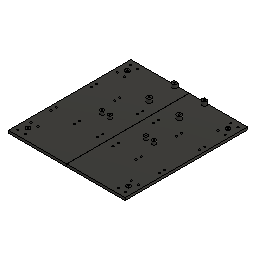
base_plate (Autodesk Fusion 360 design; units mm, degrees)
Autodesk Fusion 360 part; units mm, degrees
note: some values were not read from the file. Set by a fixed rule: which sketch regions a step uses.
sketch "Skizze2" plane through (0, 0, 0) normal (0, 0, 1) x (1, 0, 0)
  line L0 (0, 153.3528) -> (0, -137.2618) construction
  line L1 (-213.5725, 0) -> (204.3079, 0) construction
  line L2 (113.137, -118.8) -> (-113.137, -118.8)
  line L3 (-113.137, -118.8) -> (-113.137, 118.8)
  line L4 (-113.137, 118.8) -> (113.137, 118.8)
  line L5 (113.137, 118.8) -> (113.137, -118.8)
  line L6 (113.137, -118.8) -> (-113.137, 118.8) construction
  line L7 (-113.137, -118.8) -> (113.137, 118.8) construction
  line L8 (0, 118.8) -> (0, -118.8)
  line L9 (-140.8962, -96.5) -> (185.8278, -96.5) construction
  line L10 (-143.9931, -39) -> (195.1185, -39) construction
  line L11 (97.637, 133.9785) -> (97.637, -173.5851) construction
  line L12 (104.637, -109) -> (90.637, -109) construction
  line L13 (90.637, -109) -> (90.637, -84) construction
  line L14 (90.637, -84) -> (104.637, -84) construction
  line L15 (104.637, -84) -> (104.637, -109) construction
  line L16 (104.637, -109) -> (90.637, -84) construction
  line L17 (90.637, -109) -> (104.637, -84) construction
  circle A0 centre (104.637, -84) radius 1.75
  circle A1 centre (104.637, -84) radius 3.5
  circle A2 centre (90.637, -84) radius 1.75
  circle A3 centre (90.637, -84) radius 3.5
  circle A4 centre (90.637, -109) radius 1.75
  circle A5 centre (90.637, -109) radius 3.5
  circle A6 centre (104.637, -109) radius 1.75
  circle A7 centre (104.637, -109) radius 3.5
  circle A8 centre (-90.637, -109) radius 3.5
  circle A9 centre (-90.637, -109) radius 1.75
  circle A10 centre (-104.637, -109) radius 3.5
  circle A11 centre (-104.637, -109) radius 1.75
  circle A12 centre (-104.637, -84) radius 3.5
  circle A13 centre (-104.637, -84) radius 1.75
  circle A14 centre (-90.637, -84) radius 3.5
  circle A15 centre (-90.637, -84) radius 1.75
  circle A16 centre (104.637, 84) radius 3.5
  circle A17 centre (104.637, 84) radius 1.75
  circle A18 centre (90.637, 84) radius 3.5
  circle A19 centre (90.637, 84) radius 1.75
  circle A20 centre (90.637, 109) radius 3.5
  circle A21 centre (90.637, 109) radius 1.75
  circle A22 centre (104.637, 109) radius 3.5
  circle A23 centre (104.637, 109) radius 1.75
  circle A24 centre (-104.637, 109) radius 3.5
  circle A25 centre (-104.637, 109) radius 1.75
  circle A26 centre (-90.637, 109) radius 3.5
  circle A27 centre (-90.637, 109) radius 1.75
  circle A28 centre (-90.637, 84) radius 3.5
  circle A29 centre (-90.637, 84) radius 1.75
  circle A30 centre (-104.637, 84) radius 3.5
  circle A31 centre (-104.637, 84) radius 1.75
  line L18 (15, -28.2196) -> (15, -51.638) construction
  circle A32 centre (15, -34) radius 1.75
  circle A33 centre (15, -44) radius 1.75
  circle A34 centre (15, -34) radius 3.5
  circle A35 centre (15, -44) radius 3.5
  circle A36 centre (-15, -34) radius 3.5
  circle A37 centre (-15, -34) radius 1.75
  circle A38 centre (-15, -44) radius 3.5
  circle A39 centre (-15, -44) radius 1.75
  circle A40 centre (60, -34) radius 3.5
  circle A41 centre (60, -34) radius 1.75
  circle A42 centre (60, -44) radius 3.5
  circle A43 centre (60, -44) radius 1.75
  circle A44 centre (105, -34) radius 3.5
  circle A45 centre (105, -34) radius 1.75
  circle A46 centre (105, -44) radius 3.5
  circle A47 centre (105, -44) radius 1.75
  circle A48 centre (-60, -44) radius 1.75
  circle A49 centre (-60, -44) radius 3.5
  circle A50 centre (-60, -34) radius 1.75
  circle A51 centre (-60, -34) radius 3.5
  circle A52 centre (-105, -44) radius 1.75
  circle A53 centre (-105, -44) radius 3.5
  circle A54 centre (-105, -34) radius 1.75
  circle A55 centre (-105, -34) radius 3.5
  circle A56 centre (105, 44) radius 3.5
  circle A57 centre (105, 34) radius 3.5
  circle A58 centre (105, 34) radius 1.75
  circle A59 centre (60, 44) radius 3.5
  circle A60 centre (60, 44) radius 1.75
  circle A61 centre (60, 34) radius 3.5
  circle A62 centre (60, 34) radius 1.75
  circle A63 centre (15, 44) radius 3.5
  circle A64 centre (15, 44) radius 1.75
  circle A65 centre (15, 34) radius 3.5
  circle A66 centre (15, 34) radius 1.75
  circle A67 centre (-15, 34) radius 3.5
  circle A68 centre (-15, 34) radius 1.75
  circle A69 centre (-15, 44) radius 3.5
  circle A70 centre (-15, 44) radius 1.75
  circle A71 centre (-60, 44) radius 3.5
  circle A72 centre (-60, 44) radius 1.75
  circle A73 centre (-60, 34) radius 3.5
  circle A74 centre (-60, 34) radius 1.75
  circle A75 centre (-105, 34) radius 3.5
  circle A76 centre (-105, 34) radius 1.75
  circle A77 centre (-105, 44) radius 1.75
  circle A78 centre (-105, 44) radius 3.5
  circle A79 centre (97.637, -96.5) radius 1.25
  circle A80 centre (97.637, -96.5) radius 4
  line L19 (98.9072, -98.7) -> (100.1773, -96.5)
  line L20 (100.1773, -96.5) -> (98.9072, -94.3)
  line L21 (98.9072, -94.3) -> (96.3668, -94.3)
  line L22 (96.3668, -94.3) -> (95.0967, -96.5)
  line L23 (95.0967, -96.5) -> (96.3668, -98.7)
  line L24 (96.3668, -98.7) -> (98.9072, -98.7)
  circle A81 centre (97.637, 96.5) radius 4
  line L25 (96.3668, 94.3) -> (95.0967, 96.5)
  line L26 (95.0967, 96.5) -> (96.3668, 98.7)
  line L27 (96.3668, 98.7) -> (98.9072, 98.7)
  line L28 (98.9072, 98.7) -> (100.1773, 96.5)
  line L29 (98.9072, 94.3) -> (96.3668, 94.3)
  line L30 (100.1773, 96.5) -> (98.9072, 94.3)
  circle A82 centre (97.637, 96.5) radius 1.25
  circle A83 centre (-97.637, -96.5) radius 4
  line L31 (-98.9072, -94.3) -> (-96.3668, -94.3)
  line L32 (-96.3668, -94.3) -> (-95.0967, -96.5)
  line L33 (-95.0967, -96.5) -> (-96.3668, -98.7)
  line L34 (-96.3668, -98.7) -> (-98.9072, -98.7)
  line L35 (-100.1773, -96.5) -> (-98.9072, -94.3)
  line L36 (-98.9072, -98.7) -> (-100.1773, -96.5)
  circle A84 centre (-97.637, -96.5) radius 1.25
  circle A85 centre (-97.637, 96.5) radius 4
  line L37 (-95.0967, 96.5) -> (-96.3668, 98.7)
  line L38 (-96.3668, 98.7) -> (-98.9072, 98.7)
  line L39 (-98.9072, 98.7) -> (-100.1773, 96.5)
  line L40 (-100.1773, 96.5) -> (-98.9072, 94.3)
  line L41 (-96.3668, 94.3) -> (-95.0967, 96.5)
  line L42 (-98.9072, 94.3) -> (-96.3668, 94.3)
  circle A86 centre (-97.637, 96.5) radius 1.25
  line L43 (35.103, 14.7815) -> (35.103, -12.4451) construction
  line L44 (50.103, 14.7815) -> (50.103, -11.741) construction
  circle A87 centre (35.103, 0) radius 1.25
  circle A88 centre (35.103, 0) radius 4
  circle A89 centre (50.103, 0) radius 1.25
  circle A90 centre (50.103, 0) radius 4
  line L45 (36.3732, -2.2) -> (37.6433, 0)
  line L46 (37.6433, 0) -> (36.3732, 2.2)
  line L47 (36.3732, 2.2) -> (33.8328, 2.2)
  line L48 (33.8328, 2.2) -> (32.5627, 0)
  line L49 (32.5627, 0) -> (33.8328, -2.2)
  line L50 (33.8328, -2.2) -> (36.3732, -2.2)
  line L51 (51.3732, -2.2) -> (52.6433, 0)
  line L52 (52.6433, 0) -> (51.3732, 2.2)
  line L53 (51.3732, 2.2) -> (48.8328, 2.2)
  line L54 (48.8328, 2.2) -> (47.5627, 0)
  line L55 (47.5627, 0) -> (48.8328, -2.2)
  line L56 (48.8328, -2.2) -> (51.3732, -2.2)
  circle A91 centre (-50.103, 0) radius 4
  line L57 (-51.3732, 2.2) -> (-48.8328, 2.2)
  line L58 (-48.8328, 2.2) -> (-47.5627, 0)
  line L59 (-47.5627, 0) -> (-48.8328, -2.2)
  line L60 (-48.8328, -2.2) -> (-51.3732, -2.2)
  line L61 (-52.6433, 0) -> (-51.3732, 2.2)
  line L62 (-51.3732, -2.2) -> (-52.6433, 0)
  circle A92 centre (-50.103, 0) radius 1.25
  circle A93 centre (-35.103, 0) radius 4
  line L63 (-36.3732, 2.2) -> (-33.8328, 2.2)
  line L64 (-33.8328, 2.2) -> (-32.5627, 0)
  line L65 (-32.5627, 0) -> (-33.8328, -2.2)
  line L66 (-33.8328, -2.2) -> (-36.3732, -2.2)
  line L67 (-37.6433, 0) -> (-36.3732, 2.2)
  line L68 (-36.3732, -2.2) -> (-37.6433, 0)
  circle A94 centre (-35.103, 0) radius 1.25
  line L69 (-25, 115.3) -> (33, 115.3) construction
  line L70 (33, 115.3) -> (33, 66.3) construction
  line L71 (33, 66.3) -> (-25, 66.3) construction
  line L72 (-25, 66.3) -> (-25, 115.3) construction
  circle A95 centre (-25, 115.3) radius 1.5
  line L73 (-23.4412, 112.6) -> (-21.8823, 115.3)
  line L74 (-21.8823, 115.3) -> (-23.4412, 118)
  line L75 (-23.4412, 118) -> (-26.5588, 118)
  line L76 (-26.5588, 118) -> (-28.1177, 115.3)
  line L77 (-28.1177, 115.3) -> (-26.5588, 112.6)
  line L78 (-26.5588, 112.6) -> (-23.4412, 112.6)
  arc A96 (-28.2848, 118.8) -> (-21.7152, 118.8) centre (-25, 115.3) ccw
  arc A97 (29.7152, 118.8) -> (36.2848, 118.8) centre (33, 115.3) ccw
  circle A98 centre (33, 115.3) radius 1.5
  line L79 (34.5588, 112.6) -> (36.1177, 115.3)
  line L80 (36.1177, 115.3) -> (34.5588, 118)
  line L81 (34.5588, 118) -> (31.4412, 118)
  line L82 (31.4412, 118) -> (29.8823, 115.3)
  line L83 (29.8823, 115.3) -> (31.4412, 112.6)
  line L84 (31.4412, 112.6) -> (34.5588, 112.6)
  circle A99 centre (33, 66.3) radius 4.8
  circle A100 centre (33, 66.3) radius 1.5
  circle A101 centre (-25, 66.3) radius 4.8
  circle A102 centre (-25, 66.3) radius 1.5
  line L85 (34.5588, 63.6) -> (36.1177, 66.3)
  line L86 (36.1177, 66.3) -> (34.5588, 69)
  line L87 (34.5588, 69) -> (31.4412, 69)
  line L88 (31.4412, 69) -> (29.8823, 66.3)
  line L89 (29.8823, 66.3) -> (31.4412, 63.6)
  line L90 (31.4412, 63.6) -> (34.5588, 63.6)
  line L91 (-23.4412, 63.6) -> (-21.8823, 66.3)
  line L92 (-21.8823, 66.3) -> (-23.4412, 69)
  line L93 (-23.4412, 69) -> (-26.5588, 69)
  line L94 (-26.5588, 69) -> (-28.1177, 66.3)
  line L95 (-28.1177, 66.3) -> (-26.5588, 63.6)
  line L96 (-26.5588, 63.6) -> (-23.4412, 63.6)
  circle A103 centre (105, 44) radius 1.75
  point P0 (97.637, -96.5)
  point P1 (105, 44)
  point P2 (97.637, -96.5)
  point P3 (35.103, 0)
  point P4 (50.103, 0)
  point P5 (-25, 115.3)
  point P6 (33, 115.3)
  point P7 (33, 66.3)
  point P8 (-25, 66.3)
  dimension "d117" = 113.137
  dimension "d118" = 118.8
  dimension "d121" = 39
  dimension "d122" = 96.5
  dimension "d123" = 15.5
  dimension "d124" = 14
  dimension "d125" = 25
  dimension "d126" = 3.5
  dimension "d127" = 7
  dimension "d128" = 3.5
  dimension "d129" = 7
  dimension "d130" = 3.5
  dimension "d131" = 7
  dimension "d132" = 3.5
  dimension "d133" = 7
  dimension "d134" = 15
  dimension "d135" = 3.5
  dimension "d136" = 7
  dimension "d137" = 3.5
  dimension "d138" = 7
  dimension "d141" = 90
  dimension "d142" = 0
  dimension "d145" = -90
  dimension "d146" = 0
  dimension "d147" = 2.5
  dimension "d148" = 8
  dimension "d149" = 4.4
  dimension "d150" = 5
  dimension "d151" = 5
  dimension "d152" = 35.103
  dimension "d153" = 15
  dimension "d154" = 8
  dimension "d155" = 2.5
  dimension "d156" = 8
  dimension "d157" = 2.5
  dimension "d158" = 4.4
  dimension "d159" = 4.4
  dimension "d160" = 25
  dimension "d161" = 3.5
  dimension "d162" = 58
  dimension "d163" = 49
  dimension "d166" = 3
  dimension "d167" = 5.4
  dimension "d168" = 4.8
  dimension "d169" = 4.8
  dimension "d171" = 3
  dimension "d172" = 5.4
  dimension "d173" = 3
  dimension "d175" = 9.6
  dimension "d176" = 3
  dimension "d178" = 9.6
  dimension "d179" = 5.4
  dimension "d180" = 5.4
  constraint vertical L0
  constraint horizontal L1
  constraint coincident origin L1
  constraint coincident origin L0
  constraint horizontal L2
  constraint perpendicular L2 L3
  constraint parallel L2 L4
  constraint parallel L3 L5
  constraint coincident L6 origin
  constraint coincident L7 origin
  constraint midpoint L4 L8.start
  constraint midpoint L2 L8.end
  constraint parallel L2 L9
  constraint perpendicular L0 L10
  constraint perpendicular L2 L11
  constraint horizontal L12
  constraint perpendicular L12 L13
  constraint parallel L12 L14
  constraint parallel L13 L15
  constraint coincident L16 P2
  constraint coincident L17 P2
  constraint coincident L11 P2
  constraint coincident L9 P2
  constraint coincident L14.end L15.start
  constraint concentric A0 A1
  constraint coincident L13.end L14.start
  constraint concentric A2 A3
  constraint coincident L12.end L13.start
  constraint concentric A4 A5
  constraint coincident L12.start L15.end
  constraint concentric A6 A7
  constraint symmetric L0 A0 A13
  constraint symmetric L0 A1 A12
  constraint symmetric L0 A2 A15
  constraint symmetric L0 A3 A14
  constraint symmetric L0 A4 A9
  constraint symmetric L0 A5 A8
  constraint symmetric L0 A6 A11
  constraint symmetric L0 A7 A10
  constraint symmetric L1 A0 A17
  constraint symmetric L1 A1 A16
  constraint symmetric L1 A2 A19
  constraint symmetric L1 A3 A18
  constraint symmetric L1 A4 A21
  constraint symmetric L1 A5 A20
  constraint symmetric L1 A6 A23
  constraint symmetric L1 A7 A22
  constraint symmetric L1 A8 A26
  constraint symmetric L1 A9 A27
  constraint symmetric L1 A10 A24
  constraint symmetric L1 A11 A25
  constraint symmetric L1 A12 A30
  constraint symmetric L1 A13 A31
  constraint symmetric L1 A14 A28
  constraint symmetric L1 A15 A29
  constraint perpendicular L10 L18
  constraint coincident L18 A32.centre
  constraint coincident L18 A33.centre
  constraint concentric A32 A34
  constraint concentric A33 A35
  constraint symmetric L8 A32 A37
  constraint symmetric L8 A33 A39
  constraint symmetric L8 A34 A36
  constraint symmetric L8 A35 A38
  constraint symmetric L1 A32 A66
  constraint symmetric L1 A33 A64
  constraint symmetric L1 A34 A65
  constraint symmetric L1 A35 A63
  constraint symmetric L1 A36 A67
  constraint symmetric L1 A37 A68
  constraint symmetric L1 A38 A69
  constraint symmetric L1 A39 A70
  constraint symmetric L1 A40 A61
  constraint symmetric L1 A41 A62
  constraint symmetric L1 A42 A59
  constraint symmetric L1 A43 A60
  constraint symmetric L1 A44 A57
  constraint symmetric L1 A45 A58
  constraint symmetric L1 A46 A56
  constraint symmetric L1 A46.centre P1
  constraint symmetric L1 A48 A72
  constraint symmetric L1 A49 A71
  constraint symmetric L1 A50 A74
  constraint symmetric L1 A51 A73
  constraint symmetric L1 A52 A77
  constraint symmetric L1 A53 A78
  constraint symmetric L1 A54 A76
  constraint symmetric L1 A55 A75
  constraint coincident P2 P0
  constraint horizontal L21
  constraint symmetric L1 A79 A82
  constraint symmetric L1 A80 A81
  constraint symmetric L1 L19.start L27.end
  constraint symmetric L1 L19.end L28.end
  constraint symmetric L1 L20.end L29.start
  constraint symmetric L1 L21.end L25.start
  constraint symmetric L1 L22.end L25.end
  constraint symmetric L1 L23.end L26.end
  constraint symmetric L0 A79 A84
  constraint symmetric L0 A80 A83
  constraint symmetric L0 L19.start L34.end
  constraint symmetric L0 L19.end L35.start
  constraint symmetric L0 L20.end L31.start
  constraint symmetric L0 L21.end L31.end
  constraint symmetric L0 L22.end L32.end
  constraint symmetric L0 L23.end L33.end
  constraint symmetric L0 A81 A85
  constraint symmetric L0 L25.start L41.start
  constraint symmetric L0 L25.end L37.start
  constraint symmetric L0 L26.end L37.end
  constraint symmetric L0 L27.end L38.end
  constraint symmetric L0 L28.end L39.end
  constraint symmetric L0 L29.start L40.end
  constraint symmetric L0 A82 A86
  constraint perpendicular L1 L43
  constraint perpendicular L1 L44
  constraint coincident L1 P3
  constraint coincident L43 P3
  constraint concentric A87 A88
  constraint coincident L44 P4
  constraint coincident L1 P4
  constraint concentric A89 A90
  constraint coincident P3 A87.centre
  constraint coincident P4 A89.centre
  constraint horizontal L50
  constraint horizontal L56
  constraint symmetric L0 A87 A94
  constraint symmetric L0 A88 A93
  constraint symmetric L0 A89 A92
  constraint symmetric L0 A90 A91
  constraint symmetric L0 L45.start L66.end
  constraint symmetric L0 L45.end L67.start
  constraint symmetric L0 L46.end L63.start
  constraint symmetric L0 L47.end L63.end
  constraint symmetric L0 L48.end L64.end
  constraint symmetric L0 L49.end L65.end
  constraint symmetric L0 L51.start L60.end
  constraint symmetric L0 L51.end L61.start
  constraint symmetric L0 L52.end L57.start
  constraint symmetric L0 L53.end L57.end
  constraint symmetric L0 L54.end L58.end
  constraint symmetric L0 L55.end L59.end
  constraint horizontal L69
  constraint vertical L70
  constraint horizontal L71
  constraint vertical L72
  constraint coincident P5 L69.start
  constraint horizontal L78
  constraint coincident L4 A96.start
  constraint coincident L4 A96.end
  constraint coincident L4 A97.end
  constraint coincident L4 A97.start
  constraint coincident P6 L69.end
  constraint horizontal L84
  constraint coincident P7 L70.end
  constraint concentric A99 A100
  constraint coincident P8 L71.end
  constraint concentric A101 A102
  constraint horizontal L96
  constraint horizontal L90
  constraint symmetric L1 A47 A103
  measures "d117" distance of L0 L5
  measures "d118" distance of L1 L2
  measures "d121" distance of L1 L10
  measures "d122" distance of L1 L9
  measures "d123" distance of L5 L11
  measures "d124" distance of L13 L15
  measures "d125" distance of L12 L14
  measures "d126" diameter of A0
  measures "d127" diameter of A1
  measures "d128" diameter of A2
  measures "d129" diameter of A3
  measures "d130" diameter of A6
  measures "d131" diameter of A7
  measures "d132" diameter of A4
  measures "d133" diameter of A5
  measures "d134" distance of L0 L18
  measures "d135" diameter of A32
  measures "d136" diameter of A34
  measures "d137" diameter of A33
  measures "d138" diameter of A35
  measures "d147" diameter of A79
  measures "d148" diameter of A80
  measures "d149" distance of L21 L24
  measures "d150" distance of L10 A32.centre
  measures "d151" distance of L10 A33.centre
  measures "d152" distance of L8 L43
  measures "d153" distance of L43 L44
  measures "d154" diameter of A90
  measures "d155" diameter of A89
  measures "d156" diameter of A88
  measures "d157" diameter of A87
  measures "d158" distance of L53 L56
  measures "d159" distance of L47 L50
  measures "d160" distance of L0 L72
  measures "d161" distance of L4 L69
  measures "d162" distance of L70 L72
  measures "d163" distance of L69 L71
  measures "d166" diameter of A95
  measures "d167" distance of L75 L78
  measures "d168" radius of A96
  measures "d169" radius of A97
  measures "d171" diameter of A98
  measures "d172" distance of L81 L84
  measures "d173" diameter of A102
  measures "d175" diameter of A101
  measures "d176" diameter of A100
  measures "d178" diameter of A99
  measures "d179" distance of L87 L90
  measures "d180" distance of L93 L96
extrude "Extrusion4" add sketch "Skizze2" along normal blind 5 contours L2 L3 L4 L8 A96 | L4 A96 | A8 | A10 | A12 | A14 | A24 | A26 | A28 | A30 | A36 | A38 | A49 | A51 | A53 | A55 | A67 | A69 | A71 | A73 | A75 | A78 | A83 | L31 L32 L33 L34 L35 L36 | A85 | L37 L38 L39 L40 L41 L42 | A91 | L57 L58 L59 L60 L61 L62 | A92 | A93 | L63 L64 L65 L66 L67 L68 | A94 | A95 | L73 L74 L75 L76 L77 L78 | A101 | A102 | L91 L92 L93 L94 L95 L96 makes body 1
move_face "Flächen versetzen2" offset -0.1 1 faces at (0, 39.6, 1.6667) on bodies 1
extrude "Extrusion5" add sketch "Skizze2" along normal blind 5 separate body contours L2 L4 L5 L8 A97 | L4 A97 | A1 | A3 | A5 | A7 | A16 | A18 | A20 | A22 | A34 | A35 | A40 | A42 | A44 | A46 | A56 | A57 | A59 | A61 | A63 | A65 | A80 | L19 L20 L21 L22 L23 L24 | A81 | L25 L26 L27 L28 L29 L30 | A87 | A88 | A89 | A90 | L45 L46 L47 L48 L49 L50 | L51 L52 L53 L54 L55 L56 | A98 | L79 L80 L81 L82 L83 L84 | A99 | A100 | L85 L86 L87 L88 L89 L90 makes body 2
move_face "Flächen versetzen3" offset -0.1 1 faces at (0, 39.6, 1.6667) on bodies 2
extrude "Extrusion6" cut sketch "Skizze2" along normal blind 2.5 contours A1 | A3 | A5 | A7 | A8 | A10 | A12 | A14 | A16 | A18 | A20 | A22 | A24 | A26 | A28 | A30 | A34 | A35 | A36 | A38 | A40 | A42 | A44 | A46 | A49 | A51 | A53 | A55 | A56 | A57 | A59 | A61 | A63 | A65 | A67 | A69 | A71 | A73 | A75 | A78 bodies 1 2
extrude "Extrusion7" add sketch "Skizze2" along normal blind 11 contours A88 | A90 | L45 L46 L47 L48 L49 L50 | L51 L52 L53 L54 L55 L56 | A91 | L57 L58 L59 L60 L61 L62 | A93 | L63 L64 L65 L66 L67 L68 bodies 1 2
extrude "Extrusion8" cut sketch "Skizze2" along normal blind 9 contours A87 | A89 | L45 L46 L47 L48 L49 L50 | L51 L52 L53 L54 L55 L56 | L57 L58 L59 L60 L61 L62 | A92 | L63 L64 L65 L66 L67 L68 | A94 bodies 1 2
extrude "Extrusion9" add sketch "Skizze2" along normal blind 7.2 contours L45 L46 L47 L48 L49 L50 | L51 L52 L53 L54 L55 L56 | L57 L58 L59 L60 L61 L62 | L63 L64 L65 L66 L67 L68 bodies 1 2
extrude "Extrusion10" add sketch "Skizze2" along normal blind 1 contours A87 | A89 | A92 | A94 bodies 1 2
move_face "Flächen versetzen4" offset -0.2 4 faces at (-46.1229, 0.3983, 7) (-31.1229, 0.3983, 7) (39.0831, 0.3983, 7) (54.0831, 0.3983, 7) on bodies 1 2
extrude "Extrusion20" add sketch "Skizze2" along normal blind 12 contours L4 A97 | L4 A96 | L73 L74 L75 L76 L77 L78 | L79 L80 L81 L82 L83 L84 | A99 | A101 | L85 L86 L87 L88 L89 L90 | L91 L92 L93 L94 L95 L96 bodies 1 2
extrude "Extrusion13" cut sketch "Skizze2" along normal blind 10 contours A95 | L73 L74 L75 L76 L77 L78 | A98 | L79 L80 L81 L82 L83 L84 | A100 | A102 | L85 L86 L87 L88 L89 L90 | L91 L92 L93 L94 L95 L96 bodies 1 2
extrude "Extrusion14" add sketch "Skizze2" along normal blind 7.8 contours L73 L74 L75 L76 L77 L78 | L79 L80 L81 L82 L83 L84 | L85 L86 L87 L88 L89 L90 | L91 L92 L93 L94 L95 L96 bodies 1 2
extrude "Extrusion15" add sketch "Skizze2" along normal blind 1 contours A95 | A98 | A100 | A102 bodies 1 2
extrude "Extrusion16" add sketch "Skizze2" along normal blind 6 contours A79 | A80 | L19 L20 L21 L22 L23 L24 | A81 | L25 L26 L27 L28 L29 L30 | A82 | A83 | L31 L32 L33 L34 L35 L36 | A84 | A85 | L37 L38 L39 L40 L41 L42 | A86 bodies 1 2
extrude "Extrusion17" cut sketch "Skizze2" along normal blind 6 contours A79 | A82 | A84 | A86 bodies 1 2
extrude "Extrusion18" cut sketch "Skizze2" along normal blind 4 contours L19 L20 L21 L22 L23 L24 | L25 L26 L27 L28 L29 L30 | L31 L32 L33 L34 L35 L36 | L37 L38 L39 L40 L41 L42 bodies 1 2
extrude "Extrusion19" add sketch "Skizze2" along normal blind 2.2 contours L19 L20 L21 L22 L23 L24 | L25 L26 L27 L28 L29 L30 | L31 L32 L33 L34 L35 L36 | L37 L38 L39 L40 L41 L42 bodies 1 2
equation "d118 = 124 mm - 5.2 mm"
equation "d141 = ( 2 * 45 ) * 1 mm"
equation "d145 = ( -2 * 45 ) * 1 mm"
named bodies: "base_left", "base_right"
